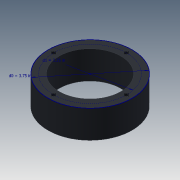
# Autodesk Inventor part: Standard
Saved by Autodesk Inventor 2020.3 (Build 243373000, 373)
## iProperties
RuleStatus: InUse
AfterDocSave0: file://Part Number Cleaner
Created: 2023-01-05
Material: ABS, BLACK
Catalog Web Link: https://www.janelia.org/
Vendor: HHMI: JRC - jET
Document SubType Name: Modeling
Designer: arnoldj
Density: 1.06 g/cm^3
Appearance: Black Anodize
DESIGN DEPARTMENT: HHMI: JRC - jET
ALTERED ITEM PART NUMBER: N/A
ALTERED ITEM VENDOR: N/A
ALTERED ITEM DESCRIPTION: N/A
Title: Standard
Author: arnoldj
Revision Number: 0
Autodesk Inventor part; units mm, degrees
ref_plane "YZ Plane" through (0, 0, 0) normal (1, 0, 0) x (0, 1, 0)
ref_plane "XZ Plane" through (0, 0, 0) normal (0, 1, 0) x (-1, 0, 0)
ref_plane "XY Plane" through (0, 0, 0) normal (0, 0, 1) x (1, 0, 0)
sketch "Sketch1" plane through (0, 0, 0) normal (0, 1, 0) x (-1, 0, 0)
  circle A0 centre (0, 0) radius 47.625
  circle A1 centre (0, 0) radius 41.275 construction
  point P0 (41.275, 0)
  point P1 (0, -41.275)
  point P2 (-41.275, 0)
  point P3 (0, 41.275)
  dimension "d0" = 95.25
  dimension "d1" = 82.55
  constraints: 4 point on circle, 2 centre point, 2 coincident
  measures "d0" diameter of A0
  measures "d1" diameter of A1
extrude "Extrusion1" add sketch "Sketch1" against normal blind 31.75
hole "Hole1" at (-41.275, 0, 0) at (0, 0, -41.275) at (41.275, 0, 0) at (0, 0, 41.275) direction (0, -1, 0) diameter 4.4958 end through all clearance for "Flat Head Machine Screw" size "M4" standard "Ansi Metric M Profile"
sketch "Sketch2" plane through (0, 0, 0) normal (0, 1, 0) x (1, 0, 0)
  point P0 (0, 0)
  point P1 (-0.2961, 4.5812)
hole "Hole2" at (0, 0, 0) direction (0, -1, 0) diameter 69.85 end through all
sketch "Sketch3" plane through (0, -31.75, 0) normal (0, -1, 0) x (1, 0, 0)
  circle A0 centre (0, 41.275) radius 2.2479 projected
  circle A1 centre (-41.275, 0) radius 2.2479 projected
  circle A2 centre (0, -41.275) radius 2.2479 projected
  circle A3 centre (41.275, 0) radius 2.2479 projected
  circle A4 centre (0, 41.275) radius 7.62
  circle A5 centre (-41.275, 0) radius 7.62
  circle A6 centre (0, -41.275) radius 7.62
  circle A7 centre (41.275, 0) radius 7.62
  point P0 (0, 0)
  dimension "d18" = 15.24
  constraints: 4 centre point, 4 coincident, 3 equal radius
  measures "d18" diameter of A4
body "Solid1"
